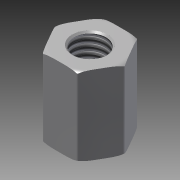
# Autodesk Inventor part: nut_rod_M3_8
Saved by Autodesk Inventor 2013 (Build 170138000, 138)
## iProperties
Shininess: 50.0
Created: 2011-05-21
Part Number: nut_rod_M3_8
Document SubType Name: Modeling
Designer: Noa Izumi
Material: Default
Density: 1 g/cm^3
Density: 0.0
Volumn: 0.0
Area: 0.0
PropertySet Name: Model Information
Control State: 0
Master: False
Checked Out: False
Author: Noa Izumi
Autodesk Inventor part; units mm, degrees
ref_plane "YZ Plane" through (0, 0, 0) normal (1, 0, 0) x (0, 1, 0)
ref_plane "XZ Plane" through (0, 0, 0) normal (0, 1, 0) x (-1, 0, 0)
ref_plane "XY Plane" through (0, 0, 0) normal (0, 0, 1) x (1, 0, 0)
sketch "Sketch1" plane through (0, 0, 0) normal (0, 0, 1) x (1, 0, 0)
  line L0 (2.6197, -0.0625) -> (1.364, -2.2375)
  line L1 (1.2557, -2.3) -> (-1.2557, -2.3)
  line L2 (-1.364, -2.2375) -> (-2.6197, -0.0625)
  line L3 (-2.6197, 0.0625) -> (-1.364, 2.2375)
  line L4 (-1.2557, 2.3) -> (1.2557, 2.3)
  line L5 (1.364, 2.2375) -> (2.6197, 0.0625)
  arc A0 (-1.2557, 2.3) -> (-1.364, 2.2375) centre (-1.2557, 2.175) ccw
  arc A1 (-2.6197, 0.0625) -> (-2.6197, -0.0625) centre (-2.5115, 0) ccw
  arc A2 (-1.364, -2.2375) -> (-1.2557, -2.3) centre (-1.2557, -2.175) ccw
  arc A3 (1.2557, -2.3) -> (1.364, -2.2375) centre (1.2557, -2.175) ccw
  arc A4 (2.6197, -0.0625) -> (2.6197, 0.0625) centre (2.5115, 0) ccw
  arc A5 (1.364, 2.2375) -> (1.2557, 2.3) centre (1.2557, 2.175) ccw
  point P0 (0, 0)
  point P1 (2.6558, 0)
  point P2 (1.3279, -2.3)
  point P3 (-1.3279, -2.3)
  point P4 (-2.6558, 0)
  point P5 (-1.3279, 2.3)
  point P6 (1.3279, 2.3)
  dimension "d36" = 4.6
  dimension "d37" = 0.125
  constraints: 12 end point, 12 point on circle, 12 point on line, 12 tangent, 6 centre point, 5 equal radius, 13 other
  measures "d36" distance between parallel lines of L1 L4
  measures "d37" radius of A0
extrude "Extrusion1" add sketch "Sketch1" along normal blind 6
sketch "草圖5" plane through (0, 0, 6) normal (0, 0, 1) x (1, 0, 0)
  point P0 (0, 0)
  point P1 (0, 0)
  constraints: 1 coincident
hole "孔2" at (0, 0, 6) direction (0, 0, -1) diameter 2.459 end through all thread size "M3x0.5" class "6H" standard "ANSI Metric M Profile"
chamfer "倒角2" distance 0.125 angle 45 2 edges at (0, 1.2295, 6) (0, 1.2295, 0)
sketch "草圖6" plane through (0, 0, 0) normal (0, 1, 0) x (-1, 0, 0)
  line L0 (-2.3, 0) -> (-2.8, 0)
  line L1 (-2.8, 6) -> (-2.3, 6)
  line L2 (-2.8, 6) -> (-2.8, 5.7)
  line L3 (-2.8, 0) -> (-2.8, 0.3)
  arc A0 (-2.3, 6) -> (-2.8, 5.7) centre (-2.3, 5.4333) ccw
  arc A1 (-2.8, 0.3) -> (-2.3, 0) centre (-2.3, 0.5667) ccw
  line L4 (0, 0) -> (0, 6)
  dimension "d48" = 6
  dimension "d50" = 2.3
  dimension "d51" = 2.3
  dimension "d52" = 0.5
  dimension "d53" = 0.3
  dimension "d54" = 0.3
  constraints: 10 end point, 4 point on circle, 2 centre point, 2 parallel, 2 tangent, 1 collinear, 1 horizontal, 1 perpendicular
  measures "d48" distance from line of L4.start L1
  measures "d50" distance of L4.start L0.start
  measures "d51" horizontal distance of L4.start L1.end
  measures "d52" distance of L1.start L1.end
  measures "d53" distance of L1.start L2.end
  measures "d54" distance of L0.end L3.end
revolve "迴轉2" cut sketch "草圖6" angle 360 about axis through (0, 0, 0) along (0, 0, 1)
